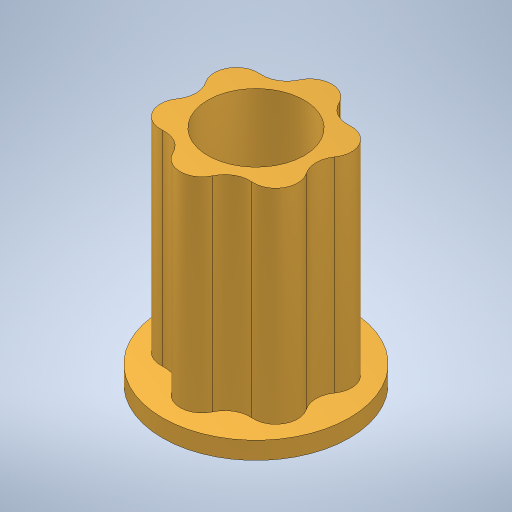
# Autodesk Inventor part: Slider
Saved by Autodesk Inventor 2023.2 (Build 272271000, 271)
## iProperties
Created: 2024-02-03
Part Number: Slider
Material: Brass, Soft Yellow
Document SubType Name: Modeling
Designer: Nathan Cai
Mass: 5.22 g
Surface Area: 12.5107 cm^2
Volume: 0.616293 cm^3
Density: 8.47 g/cm^3
Appearance: Brass - Satin
Author: Nathan Cai
Autodesk Inventor part; units mm, degrees
ref_plane "YZ Plane" through (0, 0, 0) normal (1, 0, 0) x (0, 1, 0)
ref_plane "XZ Plane" through (0, 0, 0) normal (0, 1, 0) x (-1, 0, 0)
ref_plane "XY Plane" through (0, 0, 0) normal (0, 0, 1) x (1, 0, 0)
sketch "Sketch1" plane through (0, 0, 0) normal (0, 1, 0) x (-1, 0, 0)
  circle A0 centre (0, 0) radius 3.175
  circle A1 centre (0, 0) radius 4.7625 construction
  circle A2 centre (0, 0) radius 7.9375 construction
  line L0 (0, 0) -> (4.7625, 0) construction
  line L1 (4.7625, -2.749631) -> (0, -5.499261)
  line L2 (0, -5.499261) -> (-4.7625, -2.749631)
  line L3 (-4.7625, -2.749631) -> (-4.7625, 2.749631)
  line L4 (-4.7625, 2.749631) -> (0, 5.499261)
  line L5 (0, 5.499261) -> (4.7625, 2.749631)
  line L6 (4.7625, 2.749631) -> (4.7625, -2.749631)
  arc A3 (4.471188, 0.916544) -> (4.179877, 0) centre (5.767377, 0) ccw
  line L7 (4.7625, 2.749631) -> (0, 0) construction
  arc A4 (4.471188, 0.916544) -> (4.549815, 2.626837) centre (3.175, 1.833087) ccw
  arc A5 (4.179877, 0) -> (4.471188, -0.916544) centre (5.767377, 0) ccw
  arc A6 (4.549815, -2.626837) -> (4.471188, -0.916544) centre (3.175, -1.833087) ccw
  arc A7 (4.549815, 2.626837) -> (3.029344, 3.413891) centre (3.175, 1.833087) ccw
  arc A8 (2.089938, 3.619879) -> (3.029344, 3.413891) centre (2.883688, 4.994695) ccw
  arc A9 (1.441844, 4.330434) -> (2.089938, 3.619879) centre (2.883688, 4.994695) ccw
  arc A10 (1.441844, 4.330434) -> (0, 5.253674) centre (0, 3.666174) ccw
  arc A11 (0, 5.253674) -> (-1.441844, 4.330434) centre (0, 3.666174) ccw
  arc A12 (-2.089938, 3.619879) -> (-1.441844, 4.330434) centre (-2.883688, 4.994695) ccw
  arc A13 (-3.029344, 3.413891) -> (-2.089938, 3.619879) centre (-2.883688, 4.994695) ccw
  arc A14 (-3.029344, 3.413891) -> (-4.549815, 2.626837) centre (-3.175, 1.833087) ccw
  arc A15 (-4.549815, 2.626837) -> (-4.471188, 0.916544) centre (-3.175, 1.833087) ccw
  arc A16 (-4.179877, 0) -> (-4.471188, 0.916544) centre (-5.767377, 0) ccw
  arc A17 (-4.471188, -0.916544) -> (-4.179877, 0) centre (-5.767377, 0) ccw
  arc A18 (-4.471188, -0.916544) -> (-4.549815, -2.626837) centre (-3.175, -1.833087) ccw
  arc A19 (-4.549815, -2.626837) -> (-3.029344, -3.413891) centre (-3.175, -1.833087) ccw
  arc A20 (-2.089938, -3.619879) -> (-3.029344, -3.413891) centre (-2.883688, -4.994695) ccw
  arc A21 (-1.441844, -4.330434) -> (-2.089938, -3.619879) centre (-2.883688, -4.994695) ccw
  arc A22 (-1.441844, -4.330434) -> (0, -5.253674) centre (0, -3.666174) ccw
  arc A23 (0, -5.253674) -> (1.441844, -4.330434) centre (0, -3.666174) ccw
  arc A24 (2.089938, -3.619879) -> (1.441844, -4.330434) centre (2.883688, -4.994695) ccw
  arc A25 (3.029344, -3.413891) -> (2.089938, -3.619879) centre (2.883688, -4.994695) ccw
  arc A26 (3.029344, -3.413891) -> (4.549815, -2.626837) centre (3.175, -1.833087) ccw
  point P0 (2.38125, -4.124446)
  point P1 (4.7625, 1.833087)
  point P2 (3.96875, 3.207902)
  point P3 (0.79375, 5.04099)
  point P4 (-0.79375, 5.04099)
  point P5 (-3.96875, 3.207902)
  point P6 (-4.7625, 1.833087)
  point P7 (-4.7625, -1.833087)
  point P8 (-3.96875, -3.207902)
  point P9 (-0.79375, -5.04099)
  point P10 (0.79375, -5.04099)
  point P11 (3.96875, -3.207902)
  point P12 (4.7625, -1.833087)
  dimension "d0" = 6.35
  dimension "d1" = 9.525
  dimension "d2" = 15.875
  dimension "d30" = 1.5875
  dimension "d31" = 1.5875
  dimension "d34" = 360
  constraints: 48 point on circle, 27 centre point, 16 end point, 4 coincident, 4 tangent, 3 point on line, 3 symmetric about line, 1 horizontal, 1 midpoint, 88 other
  measures "d0" diameter of A0
  measures "d1" diameter of A1
  measures "d2" diameter of A2
  measures "d30" radius of A3
  measures "d31" radius of A4
extrude "Extrusion1" add sketch "Sketch1" along normal blind 15.08125 contours L1 A26 A6 L6 | A26 A25 A24 A23 A22 A21 A20 A19 A18 A17 A16 A15 A14 A13 A12 A11 A10 A9 A8 A7 A4 A3 A5 A6 | L1 L2 A22 A23 | A4 A7 L5 L6 | L2 L3 A18 A19 | A10 A11 L4 L5 | L3 L4 A14 A15
sketch "Sketch2" plane through (0, 0, 0) normal (0, -1, 0) x (1, 0, 0)
  circle A0 centre (0, 0) radius 3.175 projected
  circle A1 centre (0, 0) radius 6.35
  dimension "d26" = 12.7
  constraints: 1 centre point, 1 coincident
  measures "d26" diameter of A1
extrude "Extrusion2" add sketch "Sketch2" against normal blind 1.190625
fillet "Fillet1" radius 1.5875 6 edges at (4.7625, 8.1359, 2.7496) (0, 8.1359, 5.4993) (-4.7625, 8.1359, 2.7496) (-4.7625, 8.1359, -2.7496) (0, 8.1359, -5.4993) (4.7625, 8.1359, -2.7496)
thread "Thread1" size "1/4-20 UNC" class "2B" standard "ANSI Unified Screw Threads" full length
thicken "Thicken1" operation add thickness 0.1 both sides no extend neighbours yes toward (-0.4640544, 0, -0.8858067) faces at (2.147002, 10.451042, 3.588477) (3.46181, 10.451042, 3.394463) (-1.208786, 5.820833, 4.695248) (4.40042, 5.820833, 0.807208) (-2.899273, 5.820833, 3.407271) (4.670597, 5.820833, -1.300784) (-4.584052, 5.820833, 1.101835) (1.826502, 10.451042, -3.810417) (-4.338852, 10.451042, -0.692439) (1.337809, 5.820833, -4.520822) (-4.747675, 5.820833, -1.616636) (-1.501147, 5.820833, -4.214479)
thicken "Thicken2" operation add thickness 0.1 both sides no extend neighbours yes toward (-0.9967573, 0, 0.0804666) faces at (-3.164704, 10.054167, 0.255481)
body "Solid1"
